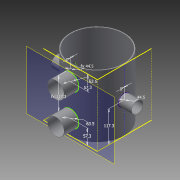
# Autodesk Inventor part: Detection Region Vacuum Collar
Saved by Autodesk Inventor 2015 (Build 190159000, 159)
## iProperties
Created: 2014-05-16
Part Number: Detection Region Vacuum Collar
Material: Generic
Document SubType Name: Modeling
Designer: ijs09
Density: 1 g/cm^3
Appearance: Default
GlobalPropertyList: <PropertyList/>
Author: ijs09
Autodesk Inventor part; units mm, degrees
ref_plane "XY Plane" through (0, 0, 0) normal (0, 0, 1) x (1, 0, 0)
sketch "Sketch1" plane through (0, 0, 0) normal (0, 0, 1) x (1, 0, 0)
  circle A0 centre (0, 0) radius 98.552
  circle A1 centre (0, 0) radius 101.85
  dimension "d0" = 197.104
  dimension "d1" = 203.7
  constraints: 2 centre point, 2 coincident
  measures "d0" diameter of A0
  measures "d1" diameter of A1
extrude "Extrusion1" add sketch "Sketch1" along normal blind 234.6
ref_plane "Work Plane1" through (101.85, 0, 0) normal (1, 0, 0) x (0, 1, 0)
sketch "Sketch3" plane through (101.85, 0, 0) normal (1, 0, 0) x (0, 1, 0)
  line L0 (-101.85, 0) -> (101.85, 0) construction
  line L1 (101.85, 234.6) -> (-101.85, 234.6) construction
  line L2 (-101.85, 0) -> (101.85, 0) projected
  line L3 (101.85, 234.6) -> (-101.85, 234.6) projected
  line L4 (101.85, 0) -> (101.85, 234.6) construction
  line L5 (-101.85, 0) -> (-101.85, 234.6) construction
  circle A0 centre (0, 117.3) radius 22.25
  line L6 (0, 0) -> (0, 234.6) construction
  dimension "d4" = 0
  dimension "d5" = 117.3
  dimension "d6" = 44.5
  constraints: 2 end point, 2 perpendicular, 1 centre point, 1 midpoint
  measures "d4" distance from line of L6 A0.centre
  measures "d5" distance from line of A0.centre L0
  measures "d6" diameter of A0
extrude "Extrusion2" add sketch "Sketch3" along normal blind 49.59
extrude "Extrusion7" add sketch "Sketch3" against normal up to next
ref_plane "Work Plane2" through (-101.85, 0, 0) normal (1, 0, 0) x (0, 1, 0)
sketch "Sketch6" plane through (-101.85, 0, 0) normal (1, 0, 0) x (0, 1, 0)
  circle A0 centre (0, 117.3) radius 22.25
  line L0 (0, 17.3) -> (0, 217.3) construction
  line L1 (-101.85, 0) -> (101.85, 0) projected
  dimension "d16" = 0
  dimension "d18" = 44.5
  dimension "d48" = 117.3
  constraints: 2 end point, 1 centre point
  measures "d16" distance from line of L0 A0.centre
  measures "d18" diameter of A0
  measures "d48" distance from line of A0.centre L1
extrude "Extrusion5" add sketch "Sketch6" against normal blind 49.59
extrude "Extrusion8" add sketch "Sketch6" along normal up to next
hole "Hole2" at (151.44, 0, 117.3) direction (-1, 0, 0) diameter 42.5 end through all
ref_plane "Work Plane3" through (0, -101.85, 0) normal (0, 1, 0) x (-1, 0, 0)
sketch "Sketch8" plane through (0, -101.85, 0) normal (0, 1, 0) x (-1, 0, 0)
  circle A0 centre (0, 57.3) radius 31.75
  circle A1 centre (0, 177.3) radius 31.75
  line L0 (-101.85, 0) -> (101.85, 0) projected
  line L1 (101.85, 234.6) -> (-101.85, 234.6) projected
  point P0 (0, 0)
  dimension "d49" = 63.5
  dimension "d50" = 63.5
  dimension "d51" = 57.3
  dimension "d75" = 57.3
  constraints: 2 centre point
  measures "d49" diameter of A0
  measures "d50" diameter of A1
  measures "d51" distance from line of A0.centre L0
  measures "d75" distance from line of A1.centre L1
extrude "Extrusion9" add sketch "Sketch8" against normal blind 54.7
extrude "Extrusion10" add sketch "Sketch8" along normal up to next
hole "Hole3" at (0, -156.55, 177.3) direction (0, 1, 0) diameter 61.7 depth 100
hole "Hole4" at (0, -156.55, 57.3) direction (0, 1, 0) diameter 61.7 depth 100
equation "\"d18\" = d6"
equation "\"d48\" = d5"
body "Solid1"
